Autodesk Inventor part; units mm, degrees
(part 2 of 3)
  arc A319 (924.0536, 1341.468) -> (949.0871, 1319.5117) centre (949.0871, 1344.7609) ccw
  line L340 (949.0871, 1319.5117) -> (1083.5982, 1319.5117)
  circle A320 centre (909.1817, 1339.5117) radius 2.5
  arc A321 (924.0536, 1341.468) -> (894.7407, 1335.4547) centre (909.1817, 1339.5117) ccw
  arc A322 (894.7407, 1335.4547) -> (955.3696, 1289.5117) centre (955.3696, 1352.4877) ccw
  arc A323 (1107.6597, 1090.5871) -> (1106.3199, 1085.5871) centre (1116.3199, 1085.5871) ccw
  arc A324 (1091.6597, 1090.5871) -> (1090.3199, 1085.5871) centre (1100.3199, 1085.5871) ccw
  arc A325 (1090.3199, 1000.9461) -> (1091.6597, 995.9461) centre (1100.3199, 1000.9461) ccw
  arc A326 (1106.3199, 1000.9461) -> (1107.6597, 995.9461) centre (1116.3199, 1000.9461) ccw
  arc A327 (1172.8199, 918.2666) -> (1187.8199, 933.2666) centre (1172.8199, 933.2666) ccw
  arc A328 (887.8199, 933.2666) -> (902.8199, 918.2666) centre (902.8199, 933.2666) ccw
  arc A329 (893.2487, 1002.5412) -> (887.8199, 990.9917) centre (902.8199, 990.9917) ccw
  arc A330 (887.8199, 1095.5415) -> (893.2487, 1083.9921) centre (902.8199, 1095.5415) ccw
  arc A331 (902.8199, 1168.2666) -> (887.8199, 1153.2666) centre (902.8199, 1153.2666) ccw
  arc A332 (1187.8199, 1153.2666) -> (1172.8199, 1168.2666) centre (1172.8199, 1153.2666) ccw
  arc A333 (1182.3912, 1083.9921) -> (1187.8199, 1095.5415) centre (1172.8199, 1095.5415) ccw
  arc A334 (1187.8199, 990.9917) -> (1182.3912, 1002.5412) centre (1172.8199, 990.9917) ccw
  arc A335 (983.9802, 995.9461) -> (985.3199, 1000.9461) centre (975.3199, 1000.9461) ccw
  arc A336 (985.3199, 1085.5871) -> (983.9802, 1090.5871) centre (975.3199, 1085.5871) ccw
  arc A337 (969.3199, 1085.5871) -> (967.9802, 1090.5871) centre (959.3199, 1085.5871) ccw
  arc A338 (967.9802, 995.9461) -> (969.3199, 1000.9461) centre (959.3199, 1000.9461) ccw
  line L341 (1091.6597, 995.9461) -> (1114.1039, 957.0716)
  line L342 (967.9802, 995.9461) -> (949.536, 963.9998)
  line L343 (1187.8199, 1153.2666) -> (1187.8199, 1095.5415)
  circle A339 centre (1007.8199, 1013.2666) radius 2.5
  circle A340 centre (1007.8199, 973.2666) radius 2.5
  circle A341 centre (987.8199, 933.2666) radius 4
  circle A342 centre (1087.8199, 933.2666) radius 4
  circle A343 centre (1067.8199, 973.2666) radius 2.5
  circle A344 centre (1067.8199, 1013.2666) radius 2.5
  arc A345 (949.536, 963.9998) -> (961.536, 957.0716) centre (955.536, 960.5357) ccw
  line L344 (983.9802, 995.9461) -> (961.536, 957.0716)
  line L345 (985.3199, 1085.5871) -> (985.3199, 1000.9461)
  line L346 (983.9802, 1090.5871) -> (961.536, 1129.4617)
  arc A346 (961.536, 1129.4617) -> (949.536, 1122.5335) centre (955.536, 1125.9976) ccw
  line L347 (967.9802, 1090.5871) -> (949.536, 1122.5335)
  line L348 (969.3199, 1085.5871) -> (969.3199, 1000.9461)
  spline S12 degree 2 poles (1157.8199, 1043.2666) (1157.8199, 1063.6293) (1182.3912, 1083.9921) knots 0.5 0.5 0.5 0.952505 0.952505 0.952505
  line L349 (1157.8199, 1043.2666) -> (1157.8199, 1063.6293) construction
  line L350 (1157.8199, 1063.6293) -> (1182.3912, 1083.9921) construction
  spline S13 degree 2 poles (1182.3912, 1002.5412) (1157.8199, 1022.9039) (1157.8199, 1043.2666) knots 0.047495 0.047495 0.047495 0.5 0.5 0.5
  line L351 (1182.3912, 1002.5412) -> (1157.8199, 1022.9039) construction
  line L352 (1157.8199, 1022.9039) -> (1157.8199, 1043.2666) construction
  line L353 (1187.8199, 990.9917) -> (1187.8199, 933.2666)
  line L354 (902.8199, 918.2666) -> (1172.8199, 918.2666)
  line L355 (887.8199, 990.9917) -> (887.8199, 933.2666)
  spline S14 degree 2 poles (893.2487, 1002.5412) (917.8199, 1022.9039) (917.8199, 1043.2666) knots 0.047495 0.047495 0.047495 0.5 0.5 0.5
  line L356 (893.2487, 1002.5412) -> (917.8199, 1022.9039) construction
  line L357 (917.8199, 1022.9039) -> (917.8199, 1043.2666) construction
  spline S15 degree 2 poles (917.8199, 1043.2666) (917.8199, 1063.6293) (893.2487, 1083.9921) knots 0.5 0.5 0.5 0.952505 0.952505 0.952505
  line L358 (917.8199, 1043.2666) -> (917.8199, 1063.6293) construction
  line L359 (917.8199, 1063.6293) -> (893.2487, 1083.9921) construction
  line L360 (887.8199, 1153.2666) -> (887.8199, 1095.5415)
  line L361 (902.8199, 1168.2666) -> (1172.8199, 1168.2666)
  arc A347 (1114.1039, 957.0716) -> (1126.1039, 963.9998) centre (1120.1039, 960.5357) ccw
  line L362 (1107.6597, 995.9461) -> (1126.1039, 963.9998)
  line L363 (1106.3199, 1085.5871) -> (1106.3199, 1000.9461)
  line L364 (1107.6597, 1090.5871) -> (1126.1039, 1122.5335)
  arc A348 (1126.1039, 1122.5335) -> (1114.1039, 1129.4617) centre (1120.1039, 1125.9976) ccw
  line L365 (1091.6597, 1090.5871) -> (1114.1039, 1129.4617)
  line L366 (1090.3199, 1085.5871) -> (1090.3199, 1000.9461)
  arc A349 (1483.1425, 925.2202) -> (1526.4438, 950.2202) centre (1504.7931, 937.7202) ccw
  arc A350 (1453.0592, 977.326) -> (1423.7771, 1006.608) centre (1383.7771, 937.326) ccw
  arc A351 (1405.0015, 1017.4482) -> (1325.0015, 1017.4482) centre (1365.0015, 948.1661) ccw
  arc A352 (1306.2258, 1006.608) -> (1276.9438, 977.326) centre (1346.2258, 937.326) ccw
  arc A353 (1203.5592, 950.2202) -> (1246.8605, 925.2202) centre (1225.2098, 937.7202) ccw
  arc A354 (1269.6232, 1043.2106) -> (1240.3412, 1013.9285) centre (1309.6232, 973.9285) ccw
  arc A355 (1289.0015, 1054.3986) -> (1329.0015, 1123.6806) centre (1249.0015, 1123.6806) ccw
  arc A356 (1401.0015, 1123.6806) -> (1441.0015, 1054.3986) centre (1481.0015, 1123.6806) ccw
  arc A357 (1489.6617, 1013.9285) -> (1460.3797, 1043.2106) centre (1420.3797, 973.9285) ccw
  circle A358 centre (1365.0015, 1133.1661) radius 2.5
  circle A359 centre (1365.0015, 1073.1661) radius 2.5
  line L367 (1240.3412, 1013.9285) -> (1203.5592, 950.2202)
  line L368 (1289.0015, 1054.3986) -> (1269.6232, 1043.2106)
  line L369 (1329.0015, 1217.4926) -> (1329.0015, 1123.6806)
  line L370 (1329.0015, 1217.4926) -> (1401.0015, 1217.4926)
  line L371 (1401.0015, 1217.4926) -> (1401.0015, 1123.6806)
  line L372 (1441.0015, 1054.3986) -> (1460.3797, 1043.2106)
  line L373 (1489.6617, 1013.9285) -> (1526.4438, 950.2202)
  line L374 (1483.1425, 925.2202) -> (1453.0592, 977.326)
  line L375 (1423.7771, 1006.608) -> (1405.0015, 1017.4482)
  line L376 (1306.2258, 1006.608) -> (1325.0015, 1017.4482)
  line L377 (1246.8605, 925.2202) -> (1276.9438, 977.326)
  arc A360 (1451.8925, 1190.3069) -> (1461.4756, 1197.4498) centre (1451.8925, 1200.3069) ccw
  arc A361 (1462.6414, 1200.5792) -> (1461.4756, 1197.4498) centre (1485.4335, 1190.3069) ccw
  line L378 (1464.6979, 1199.3919) -> (1462.6414, 1200.5792)
  arc A362 (1464.6979, 1199.3919) -> (1467.1979, 1203.722) centre (1465.9479, 1201.5569) ccw
  line L379 (1467.1979, 1203.722) -> (1465.1414, 1204.9093)
  arc A363 (1470.8311, 1210.599) -> (1465.1414, 1204.9093) centre (1485.4335, 1190.3069) ccw
  line L380 (1472.0184, 1208.5425) -> (1470.8311, 1210.599)
  arc A364 (1472.0184, 1208.5425) -> (1476.3486, 1211.0425) centre (1474.1835, 1209.7925) ccw
  line L381 (1476.3486, 1211.0425) -> (1475.1612, 1213.099)
  arc A365 (1482.9335, 1215.1816) -> (1475.1612, 1213.099) centre (1485.4335, 1190.3069) ccw
  line L382 (1482.9335, 1212.8069) -> (1482.9335, 1215.1816)
  arc A366 (1482.9335, 1212.8069) -> (1487.9335, 1212.8069) centre (1485.4335, 1212.8069) ccw
  line L383 (1487.9335, 1212.8069) -> (1487.9335, 1215.1816)
  arc A367 (1495.7058, 1213.099) -> (1487.9335, 1215.1816) centre (1485.4335, 1190.3069) ccw
  line L384 (1494.5184, 1211.0425) -> (1495.7058, 1213.099)
  arc A368 (1494.5184, 1211.0425) -> (1498.8486, 1208.5425) centre (1496.6835, 1209.7925) ccw
  line L385 (1498.8486, 1208.5425) -> (1500.0359, 1210.599)
  arc A369 (1505.7256, 1204.9093) -> (1500.0359, 1210.599) centre (1485.4335, 1190.3069) ccw
  line L386 (1503.6691, 1203.722) -> (1505.7256, 1204.9093)
  arc A370 (1503.6691, 1203.722) -> (1506.1691, 1199.3919) centre (1504.9191, 1201.5569) ccw
  line L387 (1506.1691, 1199.3919) -> (1508.2256, 1200.5792)
  arc A371 (1508.3464, 1180.3069) -> (1508.2256, 1200.5792) centre (1485.4335, 1190.3069) ccw
  line L388 (1430.4335, 1180.3069) -> (1508.3464, 1180.3069)
  arc A372 (1440.4335, 1190.3069) -> (1430.4335, 1180.3069) centre (1440.4335, 1180.3069) ccw
  line L389 (1440.4335, 1190.3069) -> (1451.8925, 1190.3069)
  circle A373 centre (1485.4335, 1190.3069) radius 2.5
  line L390 (1132.5734, 845.234) -> (1132.147, 845.234)
  line L391 (1126.5734, 727.9006) -> (1126.5734, 839.234)
  line L392 (1138.9068, 666.234) -> (1138.9068, 715.9006)
  line L393 (1144.9068, 906.9006) -> (1478.2401, 906.9006)
  line L394 (1484.2401, 715.9006) -> (1484.2401, 666.234)
  line L395 (1484.2401, 900.9006) -> (1484.2401, 851.234)
  line L396 (1138.9068, 851.9938) -> (1138.9068, 900.9006)
  line L397 (1478.2401, 660.234) -> (1144.9068, 660.234)
  line L398 (1490.2401, 845.234) -> (1490.5734, 845.234)
  line L399 (1132.9068, 721.9006) -> (1132.5734, 721.9006)
  line L400 (1496.5734, 839.234) -> (1496.5734, 727.9006)
  line L401 (1490.5734, 721.9006) -> (1490.2401, 721.9006)
  arc A374 (1132.5734, 845.234) -> (1128.6945, 843.8115) centre (1132.5734, 839.234) ccw
  arc A375 (1128.6945, 843.8115) -> (1131.5735, 840.2481) centre (1149.6563, 857.8027) ccw
  spline S16 degree 3 poles (1491.5734, 777.0673) (1491.5752, 777.0688) (1491.6024, 777.0934) (1493.9337, 779.6593) (1494.6631, 781.8259) (1494.9067, 783.7214) (1494.6, 785.5737) (1493.66, 787.851) (1491.6014, 790.041) (1491.5752, 790.0656) (1491.5734, 790.0673) knots 0 0 0 0 0.01236 0.196358 0.365814 0.504316 0.642688 0.817015 0.98764 1 1 1 1
  line L402 (1491.5734, 777.0673) -> (1491.5752, 777.0688) construction
  line L403 (1491.5752, 777.0688) -> (1491.6024, 777.0934) construction
  line L404 (1491.6024, 777.0934) -> (1493.9337, 779.6593) construction
  line L405 (1493.9337, 779.6593) -> (1494.6631, 781.8259) construction
  line L406 (1494.6631, 781.8259) -> (1494.9067, 783.7214) construction
  line L407 (1494.9067, 783.7214) -> (1494.6, 785.5737) construction
  line L408 (1494.6, 785.5737) -> (1493.66, 787.851) construction
  line L409 (1493.66, 787.851) -> (1491.6014, 790.041) construction
  line L410 (1491.6014, 790.041) -> (1491.5752, 790.0656) construction
  line L411 (1491.5752, 790.0656) -> (1491.5734, 790.0673) construction
  arc A376 (1128.6945, 843.8115) -> (1126.5734, 839.234) centre (1132.5734, 839.234) ccw
  spline S17 degree 3 poles (1131.5734, 777.0673) (1131.5717, 777.069) (1131.5455, 777.0936) (1129.4869, 779.2836) (1128.5469, 781.5609) (1128.2402, 783.4132) (1128.4838, 785.3087) (1129.2132, 787.4753) (1131.5445, 790.0412) (1131.5717, 790.0658) (1131.5734, 790.0673) knots 0 0 0 0 0.01236 0.182985 0.357312 0.495684 0.634186 0.803642 0.98764 1 1 1 1
  line L412 (1131.5734, 777.0673) -> (1131.5717, 777.069) construction
  line L413 (1131.5717, 777.069) -> (1131.5455, 777.0936) construction
  line L414 (1131.5455, 777.0936) -> (1129.4869, 779.2836) construction
  line L415 (1129.4869, 779.2836) -> (1128.5469, 781.5609) construction
  line L416 (1128.5469, 781.5609) -> (1128.2402, 783.4132) construction
  line L417 (1128.2402, 783.4132) -> (1128.4838, 785.3087) construction
  line L418 (1128.4838, 785.3087) -> (1129.2132, 787.4753) construction
  line L419 (1129.2132, 787.4753) -> (1131.5445, 790.0412) construction
  line L420 (1131.5445, 790.0412) -> (1131.5717, 790.0658) construction
  line L421 (1131.5717, 790.0658) -> (1131.5734, 790.0673) construction
  arc A377 (1132.147, 845.234) -> (1138.9068, 851.9938) centre (1132.147, 851.9938) ccw
  arc A378 (1126.5734, 727.9006) -> (1132.5734, 721.9006) centre (1132.5734, 727.9006) ccw
  circle A379 centre (1131.5734, 783.5673) radius 1.5
  arc A380 (1138.9068, 666.234) -> (1144.9068, 660.234) centre (1144.9068, 666.234) ccw
  arc A381 (1484.2401, 851.234) -> (1490.2401, 845.234) centre (1490.2401, 851.234) ccw
  arc A382 (1478.2401, 660.234) -> (1484.2401, 666.234) centre (1478.2401, 666.234) ccw
  circle A383 centre (1491.5734, 783.5673) radius 1.5
  arc A384 (1138.9068, 715.9006) -> (1132.9068, 721.9006) centre (1132.9068, 715.9006) ccw
  arc A385 (1484.2401, 900.9006) -> (1478.2401, 906.9006) centre (1478.2401, 900.9006) ccw
  arc A386 (1144.9068, 906.9006) -> (1138.9068, 900.9006) centre (1144.9068, 900.9006) ccw
  arc A387 (1496.5734, 839.234) -> (1490.5734, 845.234) centre (1490.5734, 839.234) ccw
  arc A388 (1490.2401, 721.9006) -> (1484.2401, 715.9006) centre (1490.2401, 715.9006) ccw
  arc A389 (1490.5734, 721.9006) -> (1496.5734, 727.9006) centre (1490.5734, 727.9006) ccw
  line L422 (1546.9519, 910.8763) -> (1783.6186, 910.8763)
  line L423 (1783.6186, 1300.8763) -> (1546.9519, 1300.8763)
  line L424 (1788.6186, 915.8763) -> (1788.6186, 1295.8763)
  line L425 (1541.9519, 1295.8763) -> (1541.9519, 915.8763)
  arc A390 (1541.9519, 915.8802) -> (1546.9528, 910.8763) centre (1546.9519, 915.8763) ccw
  arc A391 (1783.6146, 910.8763) -> (1788.6186, 915.8759) centre (1783.6186, 915.8763) ccw
  arc A392 (1788.6186, 1295.8735) -> (1783.619, 1300.8763) centre (1783.6186, 1295.8763) ccw
  arc A393 (1546.9559, 1300.8763) -> (1541.9519, 1295.8767) centre (1546.9519, 1295.8763) ccw
  line L426 (1712.0906, 898.4059) -> (1594.9376, 898.4059)
  circle A394 centre (1672.0141, 873.2868) radius 1.5
  circle A395 centre (1672.0141, 838.0487) radius 1.5
  circle A396 centre (1635.0141, 838.0487) radius 1.5
  circle A397 centre (1635.0141, 855.6678) radius 1.5
  circle A398 centre (1635.0141, 873.2868) radius 1.5
  circle A399 centre (1672.0141, 855.6678) radius 1.5
  line L427 (1538.2709, 775.0725) -> (1768.7572, 775.0725)
  line L428 (1590.4654, 895.6419) -> (1533.7988, 782.3086)
  line L429 (1773.2294, 782.3086) -> (1716.5627, 895.6419)
  arc A400 (1533.804, 782.319) -> (1538.2765, 775.0725) centre (1538.2709, 780.0725) ccw
  arc A401 (1768.7456, 775.0726) -> (1773.2269, 782.3136) centre (1768.7572, 780.0725) ccw
  arc A402 (1594.9412, 898.4059) -> (1590.465, 895.641) centre (1594.9376, 893.4059) ccw
  arc A403 (1716.5643, 895.6387) -> (1712.0895, 898.4059) centre (1712.0906, 893.4059) ccw
  circle A404 centre (1266.6999, 532.0426) radius 2.5
  line L430 (1279.1999, 545.0426) -> (1254.1999, 545.0426)
  line L431 (1298.6999, 517.0426) -> (1279.1999, 545.0426)
  line L432 (1234.6999, 517.0426) -> (1298.6999, 517.0426)
  line L433 (1254.1999, 545.0426) -> (1234.6999, 517.0426)
  circle A405 centre (1262.5979, 572.3835) radius 2.5
  line L434 (1275.0979, 585.3835) -> (1250.0979, 585.3835)
  line L435 (1294.5979, 557.3835) -> (1275.0979, 585.3835)
  line L436 (1230.5979, 557.3835) -> (1294.5979, 557.3835)
  line L437 (1250.0979, 585.3835) -> (1230.5979, 557.3835)
  line L438 (1478.6057, 321.2601) -> (1289.2797, 321.2601)
  line L439 (1289.2797, 321.2601) -> (1276.5158, 346.7879)
  arc A406 (1285.4601, 361.2601) -> (1276.5158, 346.7879) centre (1285.4601, 351.2601) ccw
  line L440 (1285.4601, 361.2601) -> (1452.4254, 361.2601)
  arc A407 (1461.3697, 355.7322) -> (1452.4254, 361.2601) centre (1452.4254, 351.2601) ccw
  line L441 (1478.6057, 321.2601) -> (1461.3697, 355.7322)
  circle A408 centre (1446.6057, 336.2601) radius 2.5
  arc A409 (1291.5581, 350.3172) -> (1290.9825, 349.6625) centre (1291.4834, 349.8025) ccw
  line L442 (1295.6564, 349.7224) -> (1291.5581, 350.3172)
  arc A410 (1296.9453, 346.2054) -> (1295.6564, 349.7224) centre (1295.3507, 347.6157) ccw
  arc A411 (1296.9453, 346.2054) -> (1291.3209, 338.0535) centre (1300.8803, 337.4742) ccw
  arc A412 (1291.3209, 338.0535) -> (1296.9453, 329.9983) centre (1299.9913, 338.1162) ccw
  arc A413 (1296.9453, 329.9983) -> (1305.8687, 328.1837) centre (1306.0871, 352.106) ccw
  arc A414 (1305.8687, 328.1837) -> (1306.891, 333.0468) centre (1306.1094, 330.6721) ccw
  line L443 (1306.891, 333.0468) -> (1297.7392, 336.0591)
  arc A415 (1299.4032, 341.4335) -> (1297.7392, 336.0591) centre (1300.5317, 338.1393) ccw
  line L444 (1299.4032, 341.4335) -> (1303.2214, 340.2911)
  arc A416 (1303.2214, 340.2911) -> (1304.9362, 345.253) centre (1303.9745, 342.8081) ccw
  line L445 (1304.9362, 345.253) -> (1303.3848, 345.8633)
  arc A417 (1303.2214, 348.5456) -> (1303.3848, 345.8633) centre (1303.9274, 347.2425) ccw
  line L446 (1303.2214, 348.5456) -> (1308.0245, 347.5175)
  arc A418 (1311.3904, 344.1533) -> (1308.0245, 347.5175) centre (1307.1077, 343.2344) ccw
  line L447 (1311.3904, 344.1533) -> (1313.4053, 334.7622)
  arc A419 (1313.4053, 334.7622) -> (1318.9088, 331.3615) centre (1317.789, 335.7027) ccw
  arc A420 (1318.9088, 331.3615) -> (1318.9088, 337.1587) centre (1318.1611, 334.2601) ccw
  line L448 (1318.9088, 337.1587) -> (1317.478, 343.8272)
  arc A421 (1317.478, 343.8272) -> (1306.7784, 353.8304) centre (1304.9362, 341.1362) ccw
  line L449 (1306.7784, 353.8304) -> (1290.0364, 356.2601)
  arc A422 (1290.0364, 356.2601) -> (1288.5231, 345.8325) centre (1289.2797, 351.0463) ccw
  arc A423 (1288.5231, 345.8325) -> (1290.9825, 349.6625) centre (1288.8821, 348.3066) ccw
  circle A424 centre (937.7745, 722.4991) radius 2.5
  circle A425 centre (1112.0678, 687.4991) radius 2.5
  circle A426 centre (897.7745, 737.3629) radius 2.5
  arc A427 (1126.1699, 692.611) -> (1062.152, 737.4991) centre (1062.152, 669.405) ccw
  arc A428 (1097.243, 684.9174) -> (1126.1699, 692.611) centre (1111.9647, 687.7931) ccw
  arc A429 (1097.243, 684.9174) -> (1067.5679, 707.4991) centre (1067.5679, 676.7099) ccw
  line L450 (933.9233, 707.4991) -> (1067.5679, 707.4991)
  arc A430 (902.6073, 759.4554) -> (927.6408, 737.4991) centre (927.6408, 762.7483) ccw
  line L451 (927.6408, 737.4991) -> (1062.152, 737.4991)
  circle A431 centre (887.7355, 757.4991) radius 2.5
  arc A432 (902.6073, 759.4554) -> (873.2945, 753.4421) centre (887.7355, 757.4991) ccw
  arc A433 (873.2945, 753.4421) -> (933.9233, 707.4991) centre (933.9233, 770.4751) ccw
  arc A434 (1089.1417, 491.362) -> (1087.8019, 486.362) centre (1097.8019, 486.362) ccw
  arc A435 (1073.1417, 491.362) -> (1071.8019, 486.362) centre (1081.8019, 486.362) ccw
  arc A436 (1071.8019, 401.721) -> (1073.1417, 396.721) centre (1081.8019, 401.721) ccw
  arc A437 (1087.8019, 401.721) -> (1089.1417, 396.721) centre (1097.8019, 401.721) ccw
  arc A438 (1154.3019, 319.0415) -> (1169.3019, 334.0415) centre (1154.3019, 334.0415) ccw
  arc A439 (869.3019, 334.0415) -> (884.3019, 319.0415) centre (884.3019, 334.0415) ccw
  arc A440 (874.7307, 403.3161) -> (869.3019, 391.7666) centre (884.3019, 391.7666) ccw
  arc A441 (869.3019, 496.3165) -> (874.7307, 484.767) centre (884.3019, 496.3165) ccw
  arc A442 (884.3019, 569.0415) -> (869.3019, 554.0415) centre (884.3019, 554.0415) ccw
  arc A443 (1169.3019, 554.0415) -> (1154.3019, 569.0415) centre (1154.3019, 554.0415) ccw
  arc A444 (1163.8732, 484.767) -> (1169.3019, 496.3165) centre (1154.3019, 496.3165) ccw
  arc A445 (1169.3019, 391.7666) -> (1163.8732, 403.3161) centre (1154.3019, 391.7666) ccw
  arc A446 (965.4622, 396.721) -> (966.8019, 401.721) centre (956.8019, 401.721) ccw
  arc A447 (966.8019, 486.362) -> (965.4622, 491.362) centre (956.8019, 486.362) ccw
  arc A448 (950.8019, 486.362) -> (949.4622, 491.362) centre (940.8019, 486.362) ccw
  arc A449 (949.4622, 396.721) -> (950.8019, 401.721) centre (940.8019, 401.721) ccw
  line L452 (1073.1417, 396.721) -> (1095.5859, 357.8465)
  line L453 (949.4622, 396.721) -> (931.018, 364.7747)
  line L454 (1169.3019, 554.0415) -> (1169.3019, 496.3165)
  circle A450 centre (989.3019, 414.0415) radius 2.5
  circle A451 centre (989.3019, 374.0415) radius 2.5
  circle A452 centre (969.3019, 334.0415) radius 4
  circle A453 centre (1069.3019, 334.0415) radius 4
  circle A454 centre (1049.3019, 374.0415) radius 2.5
  circle A455 centre (1049.3019, 414.0415) radius 2.5
  arc A456 (931.018, 364.7747) -> (943.018, 357.8465) centre (937.018, 361.3106) ccw
  line L455 (965.4622, 396.721) -> (943.018, 357.8465)
  line L456 (966.8019, 486.362) -> (966.8019, 401.721)
  line L457 (965.4622, 491.362) -> (943.018, 530.2366)
  arc A457 (943.018, 530.2366) -> (931.018, 523.3084) centre (937.018, 526.7725) ccw
  line L458 (949.4622, 491.362) -> (931.018, 523.3084)
  line L459 (950.8019, 486.362) -> (950.8019, 401.721)
  spline S18 degree 2 poles (1139.3019, 444.0415) (1139.3019, 464.4043) (1163.8732, 484.767) knots 0.5 0.5 0.5 0.952505 0.952505 0.952505
  line L460 (1139.3019, 444.0415) -> (1139.3019, 464.4043) construction
  line L461 (1139.3019, 464.4043) -> (1163.8732, 484.767) construction
  spline S19 degree 2 poles (1163.8732, 403.3161) (1139.3019, 423.6788) (1139.3019, 444.0415) knots 0.047495 0.047495 0.047495 0.5 0.5 0.5
  line L462 (1163.8732, 403.3161) -> (1139.3019, 423.6788) construction
  line L463 (1139.3019, 423.6788) -> (1139.3019, 444.0415) construction
  line L464 (1169.3019, 391.7666) -> (1169.3019, 334.0415)
  line L465 (884.3019, 319.0415) -> (1154.3019, 319.0415)
  line L466 (869.3019, 391.7666) -> (869.3019, 334.0415)
  spline S20 degree 2 poles (874.7307, 403.3161) (899.3019, 423.6788) (899.3019, 444.0415) knots 0.047495 0.047495 0.047495 0.5 0.5 0.5
  line L467 (874.7307, 403.3161) -> (899.3019, 423.6788) construction
  line L468 (899.3019, 423.6788) -> (899.3019, 444.0415) construction
  spline S21 degree 2 poles (899.3019, 444.0415) (899.3019, 464.4043) (874.7307, 484.767) knots 0.5 0.5 0.5 0.952505 0.952505 0.952505
  line L469 (899.3019, 444.0415) -> (899.3019, 464.4043) construction
  line L470 (899.3019, 464.4043) -> (874.7307, 484.767) construction
  line L471 (869.3019, 554.0415) -> (869.3019, 496.3165)
  line L472 (884.3019, 569.0415) -> (1154.3019, 569.0415)
  arc A458 (1095.5859, 357.8465) -> (1107.5859, 364.7747) centre (1101.5859, 361.3106) ccw
  line L473 (1089.1417, 396.721) -> (1107.5859, 364.7747)
  line L474 (1087.8019, 486.362) -> (1087.8019, 401.721)
  line L475 (1089.1417, 491.362) -> (1107.5859, 523.3084)
  arc A459 (1107.5859, 523.3084) -> (1095.5859, 530.2366) centre (1101.5859, 526.7725) ccw
  line L476 (1073.1417, 491.362) -> (1095.5859, 530.2366)
  line L477 (1071.8019, 486.362) -> (1071.8019, 401.721)
  arc A460 (1485.3799, 336.222) -> (1528.6812, 361.222) centre (1507.0305, 348.722) ccw
  arc A461 (1455.2966, 388.3278) -> (1426.0146, 417.6099) centre (1386.0146, 348.3278) ccw
  arc A462 (1407.2389, 428.45) -> (1327.2389, 428.45) centre (1367.2389, 359.168) ccw
  arc A463 (1308.4632, 417.6099) -> (1279.1812, 388.3278) centre (1348.4632, 348.3278) ccw
  arc A464 (1205.7966, 361.222) -> (1249.0979, 336.222) centre (1227.4472, 348.722) ccw
  arc A465 (1271.8606, 454.2124) -> (1242.5786, 424.9304) centre (1311.8606, 384.9304) ccw
  arc A466 (1291.2389, 465.4004) -> (1331.2389, 534.6825) centre (1251.2389, 534.6825) ccw
  arc A467 (1403.2389, 534.6825) -> (1443.2389, 465.4004) centre (1483.2389, 534.6825) ccw
  arc A468 (1491.8991, 424.9304) -> (1462.6171, 454.2124) centre (1422.6171, 384.9304) ccw
  circle A469 centre (1367.2389, 544.168) radius 2.5
  circle A470 centre (1367.2389, 484.168) radius 2.5
  line L478 (1242.5786, 424.9304) -> (1205.7966, 361.222)
  line L479 (1291.2389, 465.4004) -> (1271.8606, 454.2124)
  line L480 (1331.2389, 628.4944) -> (1331.2389, 534.6825)
  line L481 (1331.2389, 628.4944) -> (1403.2389, 628.4944)
  line L482 (1403.2389, 628.4944) -> (1403.2389, 534.6825)
  line L483 (1443.2389, 465.4004) -> (1462.6171, 454.2124)
  line L484 (1491.8991, 424.9304) -> (1528.6812, 361.222)
  line L485 (1485.3799, 336.222) -> (1455.2966, 388.3278)
  line L486 (1426.0146, 417.6099) -> (1407.2389, 428.45)
  line L487 (1308.4632, 417.6099) -> (1327.2389, 428.45)
  line L488 (1249.0979, 336.222) -> (1279.1812, 388.3278)
  arc A471 (1251.3081, 611.7607) -> (1260.8913, 618.9035) centre (1251.3081, 621.7607) ccw
  arc A472 (1262.0571, 622.033) -> (1260.8913, 618.9035) centre (1284.8492, 611.7607) ccw
  line L489 (1264.1136, 620.8456) -> (1262.0571, 622.033)
  arc A473 (1264.1136, 620.8456) -> (1266.6136, 625.1758) centre (1265.3636, 623.0107) ccw
  line L490 (1266.6136, 625.1758) -> (1264.5571, 626.3631)
  arc A474 (1270.2468, 632.0528) -> (1264.5571, 626.3631) centre (1284.8492, 611.7607) ccw
  line L491 (1271.4341, 629.9963) -> (1270.2468, 632.0528)
  arc A475 (1271.4341, 629.9963) -> (1275.7642, 632.4963) centre (1273.5992, 631.2463) ccw
  line L492 (1275.7642, 632.4963) -> (1274.5769, 634.5528)
  arc A476 (1282.3492, 636.6354) -> (1274.5769, 634.5528) centre (1284.8492, 611.7607) ccw
  line L493 (1282.3492, 634.2607) -> (1282.3492, 636.6354)
  arc A477 (1282.3492, 634.2607) -> (1287.3492, 634.2607) centre (1284.8492, 634.2607) ccw
  line L494 (1287.3492, 634.2607) -> (1287.3492, 636.6354)
  arc A478 (1295.1214, 634.5528) -> (1287.3492, 636.6354) centre (1284.8492, 611.7607) ccw
  line L495 (1293.9341, 632.4963) -> (1295.1214, 634.5528)
  arc A479 (1293.9341, 632.4963) -> (1298.2642, 629.9963) centre (1296.0992, 631.2463) ccw
  line L496 (1298.2642, 629.9963) -> (1299.4516, 632.0528)
  arc A480 (1305.1413, 626.3631) -> (1299.4516, 632.0528) centre (1284.8492, 611.7607) ccw
  line L497 (1303.0847, 625.1758) -> (1305.1413, 626.3631)
  arc A481 (1303.0847, 625.1758) -> (1305.5847, 620.8456) centre (1304.3347, 623.0107) ccw
  line L498 (1305.5847, 620.8456) -> (1307.6413, 622.033)
  arc A482 (1307.762, 601.7607) -> (1307.6413, 622.033) centre (1284.8492, 611.7607) ccw
  line L499 (1229.8492, 601.7607) -> (1307.762, 601.7607)
  arc A483 (1239.8492, 611.7607) -> (1229.8492, 601.7607) centre (1239.8492, 601.7607) ccw
  line L500 (1239.8492, 611.7607) -> (1251.3081, 611.7607)
  circle A484 centre (1284.8492, 611.7607) radius 2.5
  line L501 (1171.2389, 236.0505) -> (1170.8124, 236.0505)
  line L502 (1165.2389, 118.7172) -> (1165.2389, 230.0505)
  line L503 (1177.5722, 57.0505) -> (1177.5722, 106.7172)
  line L504 (1183.5722, 297.7172) -> (1516.9055, 297.7172)
  line L505 (1522.9055, 106.7172) -> (1522.9055, 57.0505)
  line L506 (1522.9055, 291.7172) -> (1522.9055, 242.0505)
  line L507 (1177.5722, 242.8103) -> (1177.5722, 291.7172)
  line L508 (1516.9055, 51.0505) -> (1183.5722, 51.0505)
  line L509 (1528.9055, 236.0505) -> (1529.2389, 236.0505)
  line L510 (1171.5722, 112.7172) -> (1171.2389, 112.7172)
  line L511 (1535.2389, 230.0505) -> (1535.2389, 118.7172)
  line L512 (1529.2389, 112.7172) -> (1528.9055, 112.7172)
  arc A485 (1171.2389, 236.0505) -> (1167.3599, 234.628) centre (1171.2389, 230.0505) ccw
  arc A486 (1167.3599, 234.628) -> (1170.239, 231.0646) centre (1188.3217, 248.6192) ccw
  spline S22 degree 3 poles (1530.2389, 167.8838) (1530.2406, 167.8854) (1530.2678, 167.91) (1532.5991, 170.4758) (1533.3285, 172.6425) (1533.5721, 174.5379) (1533.2654, 176.3902) (1532.3254, 178.6675) (1530.2668, 180.8575) (1530.2406, 180.8822) (1530.2389, 180.8838) knots 0 0 0 0 0.01236 0.196358 0.365814 0.504316 0.642688 0.817015 0.98764 1 1 1 1
  line L513 (1530.2389, 167.8838) -> (1530.2406, 167.8854) construction
  line L514 (1530.2406, 167.8854) -> (1530.2678, 167.91) construction
  line L515 (1530.2678, 167.91) -> (1532.5991, 170.4758) construction
  line L516 (1532.5991, 170.4758) -> (1533.3285, 172.6425) construction
  line L517 (1533.3285, 172.6425) -> (1533.5721, 174.5379) construction
  line L518 (1533.5721, 174.5379) -> (1533.2654, 176.3902) construction
  line L519 (1533.2654, 176.3902) -> (1532.3254, 178.6675) construction
  line L520 (1532.3254, 178.6675) -> (1530.2668, 180.8575) construction
  line L521 (1530.2668, 180.8575) -> (1530.2406, 180.8822) construction
  line L522 (1530.2406, 180.8822) -> (1530.2389, 180.8838) construction
  arc A487 (1167.3599, 234.628) -> (1165.2389, 230.0505) centre (1171.2389, 230.0505) ccw
  spline S23 degree 3 poles (1170.2389, 167.8838) (1170.2371, 167.8855) (1170.2109, 167.9102) (1168.1523, 170.1002) (1167.2123, 172.3775) (1166.9056, 174.2298) (1167.1492, 176.1252) (1167.8786, 178.2918) (1170.2099, 180.8577) (1170.2371, 180.8823) (1170.2389, 180.8838) knots 0 0 0 0 0.01236 0.182985 0.357312 0.495684 0.634186 0.803642 0.98764 1 1 1 1
  line L523 (1170.2389, 167.8838) -> (1170.2371, 167.8855) construction
  line L524 (1170.2371, 167.8855) -> (1170.2109, 167.9102) construction
  line L525 (1170.2109, 167.9102) -> (1168.1523, 170.1002) construction
  line L526 (1168.1523, 170.1002) -> (1167.2123, 172.3775) construction
  line L527 (1167.2123, 172.3775) -> (1166.9056, 174.2298) construction
  line L528 (1166.9056, 174.2298) -> (1167.1492, 176.1252) construction
  line L529 (1167.1492, 176.1252) -> (1167.8786, 178.2918) construction
  line L530 (1167.8786, 178.2918) -> (1170.2099, 180.8577) construction
  line L531 (1170.2099, 180.8577) -> (1170.2371, 180.8823) construction
  line L532 (1170.2371, 180.8823) -> (1170.2389, 180.8838) construction
  arc A488 (1170.8124, 236.0505) -> (1177.5722, 242.8103) centre (1170.8124, 242.8103) ccw
  arc A489 (1165.2389, 118.7172) -> (1171.2389, 112.7172) centre (1171.2389, 118.7172) ccw
  circle A490 centre (1170.2389, 174.3838) radius 1.5
  arc A491 (1177.5722, 57.0505) -> (1183.5722, 51.0505) centre (1183.5722, 57.0505) ccw
  arc A492 (1522.9055, 242.0505) -> (1528.9055, 236.0505) centre (1528.9055, 242.0505) ccw
  arc A493 (1516.9055, 51.0505) -> (1522.9055, 57.0505) centre (1516.9055, 57.0505) ccw
  circle A494 centre (1530.2389, 174.3838) radius 1.5
  arc A495 (1177.5722, 106.7172) -> (1171.5722, 112.7172) centre (1171.5722, 106.7172) ccw
  arc A496 (1522.9055, 291.7172) -> (1516.9055, 297.7172) centre (1516.9055, 291.7172) ccw
  arc A497 (1183.5722, 297.7172) -> (1177.5722, 291.7172) centre (1183.5722, 291.7172) ccw
  arc A498 (1535.2389, 230.0505) -> (1529.2389, 236.0505) centre (1529.2389, 230.0505) ccw
  arc A499 (1528.9055, 112.7172) -> (1522.9055, 106.7172) centre (1528.9055, 106.7172) ccw
  arc A500 (1529.2389, 112.7172) -> (1535.2389, 118.7172) centre (1529.2389, 118.7172) ccw
  line L533 (1540.5035, 368.3286) -> (1777.1701, 368.3286)
  line L534 (1777.1701, 758.3286) -> (1540.5035, 758.3286)
  line L535 (1782.1701, 373.3286) -> (1782.1701, 753.3286)
  line L536 (1535.5035, 753.3286) -> (1535.5035, 373.3286)
  arc A501 (1535.5035, 373.3326) -> (1540.5043, 368.3286) centre (1540.5035, 373.3286) ccw
  arc A502 (1777.1662, 368.3286) -> (1782.1701, 373.3282) centre (1777.1701, 373.3286) ccw
  arc A503 (1782.1701, 753.3259) -> (1777.1705, 758.3286) centre (1777.1701, 753.3286) ccw
  arc A504 (1540.5074, 758.3286) -> (1535.5035, 753.329) centre (1540.5035, 753.3286) ccw
  line L537 (1725.0565, 349.062) -> (1607.9035, 349.062)
  circle A505 centre (1684.98, 323.9429) radius 1.5
  circle A506 centre (1684.98, 288.7049) radius 1.5
  circle A507 centre (1647.98, 288.7049) radius 1.5
  circle A508 centre (1647.98, 306.3239) radius 1.5
  circle A509 centre (1647.98, 323.9429) radius 1.5
  circle A510 centre (1684.98, 306.3239) radius 1.5
  line L538 (1551.2368, 225.7287) -> (1781.7231, 225.7287)
  line L539 (1603.4314, 346.2981) -> (1546.7647, 232.9647)
  line L540 (1786.1953, 232.9647) -> (1729.5286, 346.2981)
  arc A511 (1546.7699, 232.9752) -> (1551.2424, 225.7287) centre (1551.2368, 230.7287) ccw
  arc A512 (1781.7115, 225.7287) -> (1786.1928, 232.9697) centre (1781.7231, 230.7287) ccw
  arc A513 (1607.9071, 349.062) -> (1603.4309, 346.2971) centre (1607.9035, 344.062) ccw
  arc A514 (1729.5302, 346.2949) -> (1725.0554, 349.062) centre (1725.0565, 344.062) ccw
  arc A515 (1257.0175, 2377.8448) -> (1266.6007, 2384.9877) centre (1257.0175, 2387.8448) ccw
  arc A516 (1267.7664, 2388.1171) -> (1266.6007, 2384.9877) centre (1290.5585, 2377.8448) ccw
  line L541 (1269.823, 2386.9298) -> (1267.7664, 2388.1171)
  arc A517 (1269.823, 2386.9298) -> (1272.323, 2391.2599) centre (1271.073, 2389.0948) ccw
  line L542 (1272.323, 2391.2599) -> (1270.2664, 2392.4473)
  arc A518 (1275.9561, 2398.137) -> (1270.2664, 2392.4473) centre (1290.5585, 2377.8448) ccw
  line L543 (1277.1435, 2396.0804) -> (1275.9561, 2398.137)
  arc A519 (1277.1435, 2396.0804) -> (1281.4736, 2398.5804) centre (1279.3085, 2397.3304) ccw
  line L544 (1281.4736, 2398.5804) -> (1280.2863, 2400.637)
  arc A520 (1288.0585, 2402.7195) -> (1280.2863, 2400.637) centre (1290.5585, 2377.8448) ccw
  line L545 (1288.0585, 2400.3448) -> (1288.0585, 2402.7195)
  arc A521 (1288.0585, 2400.3448) -> (1293.0585, 2400.3448) centre (1290.5585, 2400.3448) ccw
  line L546 (1293.0585, 2400.3448) -> (1293.0585, 2402.7195)
  arc A522 (1300.8308, 2400.637) -> (1293.0585, 2402.7195) centre (1290.5585, 2377.8448) ccw
  line L547 (1299.6435, 2398.5804) -> (1300.8308, 2400.637)
  arc A523 (1299.6435, 2398.5804) -> (1303.9736, 2396.0804) centre (1301.8085, 2397.3304) ccw
  line L548 (1303.9736, 2396.0804) -> (1305.1609, 2398.137)
  arc A524 (1310.8506, 2392.4473) -> (1305.1609, 2398.137) centre (1290.5585, 2377.8448) ccw
  line L549 (1308.7941, 2391.2599) -> (1310.8506, 2392.4473)
  arc A525 (1308.7941, 2391.2599) -> (1311.2941, 2386.9298) centre (1310.0441, 2389.0948) ccw
  line L550 (1311.2941, 2386.9298) -> (1313.3506, 2388.1171)
  arc A526 (1313.4714, 2367.8448) -> (1313.3506, 2388.1171) centre (1290.5585, 2377.8448) ccw
  line L551 (1235.5585, 2367.8448) -> (1313.4714, 2367.8448)
  arc A527 (1245.5585, 2377.8448) -> (1235.5585, 2367.8448) centre (1245.5585, 2367.8448) ccw
  line L552 (1245.5585, 2377.8448) -> (1257.0175, 2377.8448)
  circle A528 centre (1290.5585, 2377.8448) radius 2.5
  circle A529 centre (1443.983, 2341.764) radius 2.5
  circle A530 centre (1542.4782, 2193.7713) radius 2.5
  circle A531 centre (1426.209, 2380.5585) radius 2.5
  arc A532 (1556.0646, 2187.4142) -> (1542.5378, 2264.4224) centre (1494.388, 2216.2726) ccw
  arc A533 (1530.1699, 2202.4284) -> (1556.0646, 2187.4142) centre (1542.6132, 2194.0521) ccw
  arc A534 (1530.1699, 2202.4284) -> (1525.1542, 2239.3796) centre (1503.3829, 2217.6083) ccw
  line L553 (1430.6532, 2333.8805) -> (1525.1542, 2239.3796)
  arc A535 (1445.2481, 2392.7629) -> (1447.424, 2359.5361) centre (1465.2779, 2377.39) ccw
  line L554 (1447.424, 2359.5361) -> (1542.5378, 2264.4224)
  circle A536 centre (1433.3488, 2401.8957) radius 2.5
  arc A537 (1445.2481, 2392.7629) -> (1420.2688, 2409.2382) centre (1433.3488, 2401.8957) ccw
  arc A538 (1420.2688, 2409.2382) -> (1430.6532, 2333.8805) centre (1475.184, 2378.4113) ccw
  arc A539 (1443.7541, 1708.1852) -> (1453.3373, 1715.3281) centre (1443.7541, 1718.1852) ccw
  arc A540 (1454.503, 1718.4575) -> (1453.3373, 1715.3281) centre (1477.2951, 1708.1852) ccw
  line L555 (1456.5596, 1717.2701) -> (1454.503, 1718.4575)
  arc A541 (1456.5596, 1717.2701) -> (1459.0596, 1721.6003) centre (1457.8096, 1719.4352) ccw
  line L556 (1459.0596, 1721.6003) -> (1457.003, 1722.7876)
  arc A542 (1462.6927, 1728.4773) -> (1457.003, 1722.7876) centre (1477.2951, 1708.1852) ccw
  line L557 (1463.8801, 1726.4208) -> (1462.6927, 1728.4773)
  arc A543 (1463.8801, 1726.4208) -> (1468.2102, 1728.9208) centre (1466.0451, 1727.6708) ccw
  line L558 (1468.2102, 1728.9208) -> (1467.0229, 1730.9773)
  arc A544 (1474.7951, 1733.0599) -> (1467.0229, 1730.9773) centre (1477.2951, 1708.1852) ccw
  line L559 (1474.7951, 1730.6852) -> (1474.7951, 1733.0599)
  arc A545 (1474.7951, 1730.6852) -> (1479.7951, 1730.6852) centre (1477.2951, 1730.6852) ccw
  line L560 (1479.7951, 1730.6852) -> (1479.7951, 1733.0599)
  arc A546 (1487.5674, 1730.9773) -> (1479.7951, 1733.0599) centre (1477.2951, 1708.1852) ccw
  line L561 (1486.3801, 1728.9208) -> (1487.5674, 1730.9773)
  arc A547 (1486.3801, 1728.9208) -> (1490.7102, 1726.4208) centre (1488.5451, 1727.6708) ccw
  line L562 (1490.7102, 1726.4208) -> (1491.8975, 1728.4773)
  arc A548 (1497.5873, 1722.7876) -> (1491.8975, 1728.4773) centre (1477.2951, 1708.1852) ccw
  line L563 (1495.5307, 1721.6003) -> (1497.5873, 1722.7876)
  arc A549 (1495.5307, 1721.6003) -> (1498.0307, 1717.2701) centre (1496.7807, 1719.4352) ccw
  line L564 (1498.0307, 1717.2701) -> (1500.0873, 1718.4575)
  arc A550 (1500.208, 1698.1852) -> (1500.0873, 1718.4575) centre (1477.2951, 1708.1852) ccw
  line L565 (1422.2951, 1698.1852) -> (1500.208, 1698.1852)
  arc A551 (1432.2951, 1708.1852) -> (1422.2951, 1698.1852) centre (1432.2951, 1698.1852) ccw
  line L566 (1432.2951, 1708.1852) -> (1443.7541, 1708.1852)
  circle A552 centre (1477.2951, 1708.1852) radius 2.5
  arc A553 (1441.6475, 1125.0244) -> (1451.2307, 1132.1673) centre (1441.6475, 1135.0244) ccw
  arc A554 (1452.3964, 1135.2967) -> (1451.2307, 1132.1673) centre (1475.1885, 1125.0244) ccw
  line L567 (1454.453, 1134.1093) -> (1452.3964, 1135.2967)
  arc A555 (1454.453, 1134.1093) -> (1456.953, 1138.4395) centre (1455.703, 1136.2744) ccw
  line L568 (1456.953, 1138.4395) -> (1454.8964, 1139.6268)
  arc A556 (1460.5861, 1145.3165) -> (1454.8964, 1139.6268) centre (1475.1885, 1125.0244) ccw
  line L569 (1461.7735, 1143.26) -> (1460.5861, 1145.3165)
  arc A557 (1461.7735, 1143.26) -> (1466.1036, 1145.76) centre (1463.9385, 1144.51) ccw
  line L570 (1466.1036, 1145.76) -> (1464.9163, 1147.8165)
  arc A558 (1472.6885, 1149.8991) -> (1464.9163, 1147.8165) centre (1475.1885, 1125.0244) ccw
  line L571 (1472.6885, 1147.5244) -> (1472.6885, 1149.8991)
  arc A559 (1472.6885, 1147.5244) -> (1477.6885, 1147.5244) centre (1475.1885, 1147.5244) ccw
  line L572 (1477.6885, 1147.5244) -> (1477.6885, 1149.8991)
  arc A560 (1485.4608, 1147.8165) -> (1477.6885, 1149.8991) centre (1475.1885, 1125.0244) ccw
  line L573 (1484.2735, 1145.76) -> (1485.4608, 1147.8165)
  arc A561 (1484.2735, 1145.76) -> (1488.6036, 1143.26) centre (1486.4385, 1144.51) ccw
  line L574 (1488.6036, 1143.26) -> (1489.7909, 1145.3165)
  arc A562 (1495.4806, 1139.6268) -> (1489.7909, 1145.3165) centre (1475.1885, 1125.0244) ccw
  line L575 (1493.4241, 1138.4395) -> (1495.4806, 1139.6268)
  arc A563 (1493.4241, 1138.4395) -> (1495.9241, 1134.1093) centre (1494.6741, 1136.2744) ccw
  line L576 (1495.9241, 1134.1093) -> (1497.9806, 1135.2967)
  arc A564 (1498.1014, 1115.0244) -> (1497.9806, 1135.2967) centre (1475.1885, 1125.0244) ccw
  line L577 (1420.1885, 1115.0244) -> (1498.1014, 1115.0244)
  arc A565 (1430.1885, 1125.0244) -> (1420.1885, 1115.0244) centre (1430.1885, 1115.0244) ccw
  line L578 (1430.1885, 1125.0244) -> (1441.6475, 1125.0244)
  circle A566 centre (1475.1885, 1125.0244) radius 2.5
  arc A567 (1440.7988, 568.6369) -> (1450.3819, 575.7797) centre (1440.7988, 578.6369) ccw
  arc A568 (1451.5477, 578.9092) -> (1450.3819, 575.7797) centre (1474.3398, 568.6369) ccw
  line L579 (1453.6042, 577.7218) -> (1451.5477, 578.9092)
  arc A569 (1453.6042, 577.7218) -> (1456.1042, 582.0519) centre (1454.8542, 579.8869) ccw
  line L580 (1456.1042, 582.0519) -> (1454.0477, 583.2393)
  arc A570 (1459.7374, 588.929) -> (1454.0477, 583.2393) centre (1474.3398, 568.6369) ccw
  line L581 (1460.9247, 586.8725) -> (1459.7374, 588.929)
  arc A571 (1460.9247, 586.8725) -> (1465.2548, 589.3725) centre (1463.0898, 588.1225) ccw
  line L582 (1465.2548, 589.3725) -> (1464.0675, 591.429)
  arc A572 (1471.8398, 593.5116) -> (1464.0675, 591.429) centre (1474.3398, 568.6369) ccw
  line L583 (1471.8398, 591.1369) -> (1471.8398, 593.5116)
  arc A573 (1471.8398, 591.1369) -> (1476.8398, 591.1369) centre (1474.3398, 591.1369) ccw
  line L584 (1476.8398, 591.1369) -> (1476.8398, 593.5116)
  arc A574 (1484.6121, 591.429) -> (1476.8398, 593.5116) centre (1474.3398, 568.6369) ccw
  line L585 (1483.4247, 589.3725) -> (1484.6121, 591.429)
  arc A575 (1483.4247, 589.3725) -> (1487.7548, 586.8725) centre (1485.5898, 588.1225) ccw
  line L586 (1487.7548, 586.8725) -> (1488.9422, 588.929)
  arc A576 (1494.6319, 583.2393) -> (1488.9422, 588.929) centre (1474.3398, 568.6369) ccw
  line L587 (1492.5754, 582.0519) -> (1494.6319, 583.2393)
  arc A577 (1492.5754, 582.0519) -> (1495.0754, 577.7218) centre (1493.8254, 579.8869) ccw
  line L588 (1495.0754, 577.7218) -> (1497.1319, 578.9092)
  arc A578 (1497.2527, 558.6369) -> (1497.1319, 578.9092) centre (1474.3398, 568.6369) ccw
  line L589 (1419.3398, 558.6369) -> (1497.2527, 558.6369)
  arc A579 (1429.3398, 568.6369) -> (1419.3398, 558.6369) centre (1429.3398, 558.6369) ccw
  line L590 (1429.3398, 568.6369) -> (1440.7988, 568.6369)
  circle A580 centre (1474.3398, 568.6369) radius 2.5
  line L591 (1034.7826, 1495.3604) -> (917.6296, 1495.3604)
  circle A581 centre (994.7061, 1470.2413) radius 1.5
  circle A582 centre (994.7061, 1435.0032) radius 1.5
  circle A583 centre (957.7061, 1435.0032) radius 1.5
  circle A584 centre (957.7061, 1452.6223) radius 1.5
  circle A585 centre (957.7061, 1470.2413) radius 1.5
  circle A586 centre (994.7061, 1452.6223) radius 1.5
  line L592 (860.9629, 1372.027) -> (1091.4492, 1372.027)
  line L593 (913.1574, 1492.5964) -> (856.4908, 1379.2631)
  line L594 (1095.9214, 1379.2631) -> (1039.2547, 1492.5964)
  arc A587 (856.496, 1379.2735) -> (860.9685, 1372.027) centre (860.9629, 1377.027) ccw
  arc A588 (1091.4376, 1372.0271) -> (1095.9189, 1379.2681) centre (1091.4492, 1377.027) ccw
  arc A589 (917.6332, 1495.3604) -> (913.157, 1492.5955) centre (917.6296, 1490.3604) ccw
  arc A590 (1039.2563, 1492.5932) -> (1034.7815, 1495.3604) centre (1034.7826, 1490.3604) ccw
  line L595 (1057.5808, 911.1991) -> (940.4278, 911.1991)
  circle A591 centre (1017.5043, 886.08) radius 1.5
  circle A592 centre (1017.5043, 850.8419) radius 1.5
  circle A593 centre (980.5043, 850.8419) radius 1.5
  circle A594 centre (980.5043, 868.461) radius 1.5
  circle A595 centre (980.5043, 886.08) radius 1.5
  circle A596 centre (1017.5043, 868.461) radius 1.5
  line L596 (883.7612, 787.8657) -> (1114.2475, 787.8657)
  line L597 (935.9557, 908.4351) -> (879.289, 795.1018)
  line L598 (1118.7196, 795.1018) -> (1062.053, 908.4351)
  arc A597 (879.2943, 795.1122) -> (883.7667, 787.8657) centre (883.7612, 792.8657) ccw
  arc A598 (1114.2358, 787.8658) -> (1118.7171, 795.1068) centre (1114.2475, 792.8657) ccw
  arc A599 (940.4314, 911.1991) -> (935.9552, 908.4342) centre (940.4278, 906.1991) ccw
  arc A600 (1062.0546, 908.4319) -> (1057.5798, 911.1991) centre (1057.5808, 906.1991) ccw
  line L599 (1730.5008, 174.1106) -> (1613.3478, 174.1106)
  circle A601 centre (1690.4243, 148.9915) radius 1.5
  circle A602 centre (1690.4243, 113.7534) radius 1.5
  circle A603 centre (1653.4243, 113.7534) radius 1.5
  circle A604 centre (1653.4243, 131.3725) radius 1.5
  circle A605 centre (1653.4243, 148.9915) radius 1.5
  circle A606 centre (1690.4243, 131.3725) radius 1.5
  line L600 (1556.6811, 50.7772) -> (1787.1675, 50.7772)
  line L601 (1608.8757, 171.3466) -> (1552.209, 58.0133)
  line L602 (1791.6396, 58.0133) -> (1734.9729, 171.3466)
  arc A607 (1552.2142, 58.0237) -> (1556.6867, 50.7772) centre (1556.6811, 55.7772) ccw
  arc A608 (1787.1558, 50.7772) -> (1791.6371, 58.0183) centre (1787.1675, 55.7772) ccw
  arc A609 (1613.3514, 174.1106) -> (1608.8752, 171.3457) centre (1613.3478, 169.1106) ccw
  arc A610 (1734.9745, 171.3434) -> (1730.4998, 174.1106) centre (1730.5008, 169.1106) ccw
  circle A611 centre (958.2124, 640.9358) radius 2.5
  circle A612 centre (1132.5057, 605.9358) radius 2.5
  circle A613 centre (918.2124, 655.7996) radius 2.5
  arc A614 (1146.6077, 611.0477) -> (1082.5899, 655.9358) centre (1082.5899, 587.8417) ccw
  arc A615 (1117.6808, 603.3541) -> (1146.6077, 611.0477) centre (1132.4026, 606.2298) ccw
  arc A616 (1117.6808, 603.3541) -> (1088.0057, 625.9358) centre (1088.0057, 595.1466) ccw
  line L603 (954.3612, 625.9358) -> (1088.0057, 625.9358)
  arc A617 (923.0452, 677.8921) -> (948.0787, 655.9358) centre (948.0787, 681.185) ccw
  line L604 (948.0787, 655.9358) -> (1082.5899, 655.9358)
  circle A618 centre (908.1733, 675.9358) radius 2.5
  arc A619 (923.0452, 677.8921) -> (893.7324, 671.8788) centre (908.1733, 675.9358) ccw
  arc A620 (893.7324, 671.8788) -> (954.3612, 625.9358) centre (954.3612, 688.9118) ccw
  circle A621 centre (997.0875, 1229.8086) radius 2.5
  circle A622 centre (1171.3808, 1194.8086) radius 2.5
  circle A623 centre (957.0875, 1244.6723) radius 2.5
  arc A624 (1185.4829, 1199.9205) -> (1121.465, 1244.8086) centre (1121.465, 1176.7145) ccw
  arc A625 (1156.556, 1192.2268) -> (1185.4829, 1199.9205) centre (1171.2777, 1195.1026) ccw
  arc A626 (1156.556, 1192.2268) -> (1126.8808, 1214.8086) centre (1126.8808, 1184.0194) ccw
  line L605 (993.2363, 1214.8086) -> (1126.8808, 1214.8086)
  arc A627 (961.9203, 1266.7648) -> (986.9538, 1244.8086) centre (986.9538, 1270.0577) ccw
  line L606 (986.9538, 1244.8086) -> (1121.465, 1244.8086)
  circle A628 centre (947.0484, 1264.8086) radius 2.5
  arc A629 (961.9203, 1266.7648) -> (932.6075, 1260.7515) centre (947.0484, 1264.8086) ccw
  arc A630 (932.6075, 1260.7515) -> (993.2363, 1214.8086) centre (993.2363, 1277.7846) ccw
  circle A631 centre (939.0449, 1830.6375) radius 2.5
  circle A632 centre (1113.3382, 1795.6375) radius 2.5
  circle A633 centre (899.0449, 1845.5013) radius 2.5
  arc A634 (1127.4402, 1800.7494) -> (1063.4224, 1845.6375) centre (1063.4224, 1777.5434) ccw
  arc A635 (1098.5133, 1793.0558) -> (1127.4402, 1800.7494) centre (1113.2351, 1795.9315) ccw
  arc A636 (1098.5133, 1793.0558) -> (1068.8382, 1815.6375) centre (1068.8382, 1784.8483) ccw
  line L607 (935.1937, 1815.6375) -> (1068.8382, 1815.6375)
  arc A637 (903.8777, 1867.5938) -> (928.9112, 1845.6375) centre (928.9112, 1870.8867) ccw
  line L608 (928.9112, 1845.6375) -> (1063.4224, 1845.6375)
  circle A638 centre (889.0058, 1865.6375) radius 2.5
  arc A639 (903.8777, 1867.5938) -> (874.5649, 1861.5805) centre (889.0058, 1865.6375) ccw
  arc A640 (874.5649, 1861.5805) -> (935.1937, 1815.6375) centre (935.1937, 1878.6135) ccw
  line L609 (43.6226, 2365.5668) -> (43.6226, 2398.5668)
  line L610 (318.6226, 2365.5668) -> (318.6226, 2398.5668)
  line L611 (318.6226, 2365.5668) -> (43.6226, 2365.5668)
  circle A641 centre (200.9226, 2393.0668) radius 3
  circle A642 centre (81.3226, 2393.0668) radius 3
  line L612 (43.6226, 2398.5668) -> (43.6226, 2410.5668)
  line L613 (318.6226, 2410.5668) -> (43.6226, 2410.5668)
  line L614 (318.6226, 2398.5668) -> (318.6226, 2410.5668)
  line L615 (796.8508, 2379.0345) -> (656.8508, 2379.0345)
  arc A643 (796.8508, 2379.0345) -> (806.8508, 2389.0345) centre (796.8508, 2389.0345) ccw
  line L616 (806.8508, 2389.0345) -> (806.8508, 2400.0345)
  line L617 (846.3508, 2400.0345) -> (846.3508, 2367.0345)
  line L618 (846.3508, 2367.0345) -> (607.3508, 2367.0345)
  line L619 (607.3508, 2400.0345) -> (607.3508, 2367.0345)
  arc A644 (646.8508, 2389.0345) -> (656.8508, 2379.0345) centre (656.8508, 2389.0345) ccw
  line L620 (646.8508, 2389.0345) -> (646.8508, 2400.0345)
  line L621 (834.3508, 2412.0345) -> (806.8508, 2412.0345)
  arc A645 (846.3508, 2400.0345) -> (834.3508, 2412.0345) centre (834.3508, 2400.0345) ccw
  line L622 (37.5026, 1912.6164) -> (37.5026, 1945.6164)
  line L623 (312.5026, 1912.6164) -> (312.5026, 1945.6164)
  line L624 (312.5026, 1912.6164) -> (37.5026, 1912.6164)
  circle A646 centre (194.8026, 1940.1164) radius 3
  circle A647 centre (75.2026, 1940.1164) radius 3
  line L625 (37.5026, 1945.6164) -> (37.5026, 1957.6164)
  line L626 (312.5026, 1957.6164) -> (37.5026, 1957.6164)
  line L627 (312.5026, 1945.6164) -> (312.5026, 1957.6164)
  line L628 (790.7308, 1926.0842) -> (650.7308, 1926.0842)
  arc A648 (790.7308, 1926.0842) -> (800.7308, 1936.0842) centre (790.7308, 1936.0842) ccw
  line L629 (800.7308, 1936.0842) -> (800.7308, 1947.0842)
  line L630 (840.2308, 1947.0842) -> (840.2308, 1914.0842)
  line L631 (840.2308, 1914.0842) -> (601.2308, 1914.0842)
  line L632 (601.2308, 1947.0842) -> (601.2308, 1914.0842)
  arc A649 (640.7308, 1936.0842) -> (650.7308, 1926.0842) centre (650.7308, 1936.0842) ccw
  line L633 (640.7308, 1936.0842) -> (640.7308, 1947.0842)
  line L634 (828.2308, 1959.0842) -> (800.7308, 1959.0842)
  arc A650 (840.2308, 1947.0842) -> (828.2308, 1959.0842) centre (828.2308, 1947.0842) ccw
  line L635 (800.7308, 1947.0842) -> (800.7308, 1959.0842)
  line L636 (640.7308, 1959.0842) -> (613.2308, 1959.0842)
  arc A651 (613.2308, 1959.0842) -> (601.2308, 1947.0842) centre (613.2308, 1947.0842) ccw
  line L637 (640.7308, 1947.0842) -> (640.7308, 1959.0842)
  line L638 (312.1466, 1863.061) -> (312.1466, 1896.061)
  line L639 (37.1466, 1863.061) -> (312.1466, 1863.061)
  line L640 (37.1466, 1863.061) -> (37.1466, 1896.061)
  circle A652 centre (274.4466, 1879.561) radius 3
  circle A653 centre (154.8466, 1879.561) radius 3
  circle A654 centre (234.4466, 1890.561) radius 3
  circle A655 centre (114.8466, 1890.561) radius 3
  line L641 (312.1466, 1908.061) -> (312.1466, 1896.061)
  line L642 (37.1466, 1908.061) -> (37.1466, 1896.061)
  line L643 (37.1466, 1908.061) -> (312.1466, 1908.061)
  line L644 (594.3089, 1957.1461) -> (594.3089, 1945.1461)
  line L645 (319.3089, 1957.1461) -> (319.3089, 1945.1461)
  line L646 (319.3089, 1957.1461) -> (594.3089, 1957.1461)
  line L647 (594.3089, 1912.1461) -> (594.3089, 1945.1461)
  line L648 (319.3089, 1912.1461) -> (594.3089, 1912.1461)
  line L649 (319.3089, 1912.1461) -> (319.3089, 1945.1461)
  circle A656 centre (556.6089, 1939.6461) radius 3
  circle A657 centre (437.0089, 1939.6461) radius 3
  line L650 (319.1329, 1862.3206) -> (319.1329, 1895.3206)
  line L651 (594.1329, 1862.3206) -> (594.1329, 1895.3206)
  line L652 (594.1329, 1862.3206) -> (319.1329, 1862.3206)
  circle A658 centre (516.4329, 1889.8206) radius 3
  circle A659 centre (396.8329, 1889.8206) radius 3
  circle A660 centre (476.4329, 1878.8206) radius 3
  circle A661 centre (356.8329, 1878.8206) radius 3
  line L653 (319.1329, 1895.3206) -> (319.1329, 1907.3206)
  line L654 (594.1329, 1907.3206) -> (319.1329, 1907.3206)
  line L655 (594.1329, 1895.3206) -> (594.1329, 1907.3206)
  line L656 (793.2426, 1875.5354) -> (653.2426, 1875.5354)
  arc A662 (793.2426, 1875.5354) -> (803.2426, 1885.5354) centre (793.2426, 1885.5354) ccw
  line L657 (803.2426, 1885.5354) -> (803.2426, 1896.5354)
  line L658 (842.7426, 1896.5354) -> (842.7426, 1863.5354)
  line L659 (842.7426, 1863.5354) -> (603.7426, 1863.5354)
  line L660 (603.7426, 1896.5354) -> (603.7426, 1863.5354)